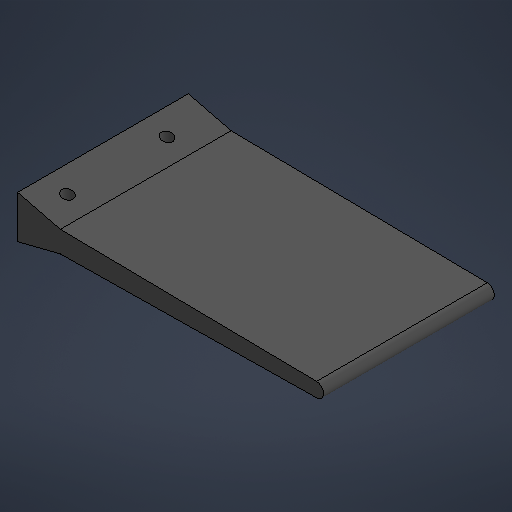
# Autodesk Inventor part: CAST,SLAB-OF-FLOP
Saved by Autodesk Inventor 2026 (Build 300175000, 175)
## iProperties
Created: 2026-02-10
Part Number: CAST,SLAB-OF-FLOP
Material: 50A Urithane
Document SubType Name: Modeling
Designer: littl
Mass: 84.7063 g
Surface Area: 250.158 cm^2
Volume: 91.0821 cm^3
Density: 1 g/cm^3
Appearance: Generic
Author: littl
Autodesk Inventor part; units mm, degrees
ref_plane "YZ Plane" through (0, 0, 0) normal (1, 0, 0) x (0, 1, 0)
ref_plane "XY Plane" through (0, 0, 0) normal (0, 0, 1) x (1, 0, 0)
sketch "Sketch1" plane through (0, 0, 0) normal (0, 0, 1) x (1, 0, 0)
  line L0 (0, 9.525) -> (0, -9.525)
  line L1 (19.05, -4.7625) -> (19.05, 4.7625) construction
  line L2 (0, 9.525) -> (19.05, 4.7625)
  line L3 (19.05, -4.7625) -> (0, -9.525)
  arc A0 (133.3941, -3.1747) -> (133.3941, 3.1747) centre (133.35, 0) ccw
  line L4 (19.05, 4.7625) -> (133.3941, 3.1747)
  line L5 (133.3941, -3.1747) -> (19.05, -4.7625)
  point P0 (0, 0)
  point P1 (19.05, 0)
  dimension "d0" = 19.05
  dimension "d1" = 9.525
  dimension "d2" = 19.05
  dimension "d3" = 3.175
  dimension "d4" = 114.3
  constraints: 12 end point, 2 horizontal alignment, 2 midpoint, 2 point on circle, 2 tangent, 2 vertical, 1 centre point
  measures "d0" distance of L0.start L0.end
  measures "d1" distance of L1.start L1.end
  measures "d2" distance between parallel lines of L0 L1
  measures "d3" radius of A0
  measures "d4" distance from line of L1 A0.centre
extrude "Extrusion1" add sketch "Sketch1" along normal blind 76.2
ref_plane "Work Plane1" through (0, 9.525, 0) normal (0, 1, 0) x (-1, 0, 0)
sketch "Sketch2" plane through (0, 9.525, 0) normal (0, 1, 0) x (-1, 0, 0)
  line L0 (-19.05, 0) -> (-19.05, 76.2) projected
  circle A0 centre (-9.525, 19.05) radius 2.54
  circle A1 centre (-9.525, 63.5) radius 2.54
  point P0 (0, 0)
  dimension "d8" = 44.45
  dimension "d9" = 19.05
  dimension "d11" = 9.525
  dimension "d12" = 5.08
  constraints: 2 centre point, 2 coincident, 1 equal radius, 1 vertical alignment
  measures "d8" distance of point (-9.525, 63.5) point (-9.525, 19.05)
  measures "d9" vertical distance of point (0, 0) point (-9.525, 19.05)
  measures "d11" distance from line of L0 point (-9.525, 19.05)
  measures "d12" diameter of A0
extrude "Extrusion2" cut sketch "Sketch2" against normal through all
body "Solid1"
